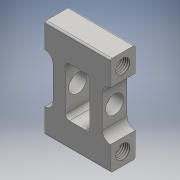
# Autodesk Inventor part: Profile_Middle_04
Saved by Autodesk Inventor 2016 (Build 200138000, 138)
## iProperties
Created: 2016-02-09
Part Number: Profile_Middle_04
Material: Generic
Document SubType Name: Modeling
Designer: nils
Density: 1 g/cm^3
Appearance: Default
Mass: 151.957 g
Surface Area: 392.667 cm^2
Volume: 151.957 cm^3
Author: nils
Autodesk Inventor part; units mm, degrees
ref_plane "YZ Plane" through (0, 0, 0) normal (1, 0, 0) x (0, 1, 0)
ref_plane "XZ Plane" through (0, 0, 0) normal (0, 1, 0) x (-1, 0, 0)
sketch "Sketch1" plane through (0, 0, 0) normal (1, 0, 0) x (0, 1, 0)
  line L0 (-15, 60) -> (15, 60)
  line L1 (15, 60) -> (15, -60)
  line L2 (15, -60) -> (-15, -60)
  line L3 (-15, -60) -> (-15, 60)
  line L4 (-15, 60) -> (15, -60) construction
  line L5 (15, 60) -> (-15, -60) construction
  point P0 (0, 0)
  dimension "d0" = 30
  dimension "d1" = 120
  constraints: 12 end point, 2 midpoint, 2 parallel, 1 horizontal, 1 perpendicular
  measures "d0" distance of L1.end L2.end
  measures "d1" distance of L0.end L1.end
extrude "Extrusion1" add sketch "Sketch1" along normal blind 80
sketch "Sketch2" plane through (80, 0, 0) normal (1, 0, 0) x (0, 0, -1)
  line L0 (-60, 15) -> (-60, -15) projected
  line L1 (-60, 0) -> (60, 0)
  line L2 (60, -15) -> (60, 15) projected
  line L3 (60, 15) -> (-60, 15) projected
  line L4 (0, 15) -> (0, -15)
  line L5 (-60, -15) -> (60, -15) projected
  point P0 (0, 0)
  point P1 (-45, 0)
  point P2 (45, 0)
  dimension "d4" = 45
  constraints: 4 end point, 4 midpoint, 2 point on line, 1 symmetric about line
  measures "d4" distance from line of L4 point (-45, 0)
hole "Hole1" at (80, 0, 45) at (80, 0, -45) direction (-1, 0, 0) diameter 17.294 depth 41.2 tip angle 118 thread size "M20x2.5" class "6H" standard "ISO Metric profile"
ref_plane "Work Plane1" through (40, 0, 0) normal (1, 0, 0) x (0, 0, -1)
mirror "Mirror1" about plane through (40, 0, 0) normal (1, 0, 0) of "Hole1"
sketch "Sketch5" plane through (0, 15, 60) normal (0, 1, 0) x (1, 0, 0)
  line L0 (0, 0) -> (80, 0) projected
  line L1 (40, 0) -> (40, 120)
  line L2 (0, 120) -> (80, 120) projected
  line L3 (55, 30) -> (25, 30)
  line L4 (25, 30) -> (25, 90)
  line L5 (25, 90) -> (55, 90)
  line L6 (55, 90) -> (55, 30)
  line L7 (55, 30) -> (25, 90) construction
  line L8 (25, 30) -> (55, 90) construction
  line L9 (0, 0) -> (0, 120) projected
  line L10 (0, 30) -> (10, 30)
  line L11 (10, 30) -> (10, 90)
  line L12 (10, 90) -> (0, 90)
  line L13 (0, 90) -> (0, 30)
  line L14 (80, 0) -> (80, 120) projected
  line L15 (80, 30) -> (70, 30)
  line L16 (70, 30) -> (70, 90)
  line L17 (70, 90) -> (80, 90)
  line L18 (80, 90) -> (80, 30)
  point P0 (0, 60)
  point P1 (40, 60)
  dimension "d20" = 30
  dimension "d22" = 30
  dimension "d23" = 30
  dimension "d24" = 60
  dimension "d25" = 10
  dimension "d26" = 10
  constraints: 30 end point, 6 parallel, 5 midpoint, 4 point on line, 3 horizontal, 3 perpendicular, 1 collinear
  measures "d20" distance between parallel lines of L0 L3
  measures "d22" distance between parallel lines of L6 L4
  measures "d23" distance between parallel lines of L2 L5
  measures "d24" distance between parallel lines of L17 L15
  measures "d25" distance between parallel lines of L18 L16
  measures "d26" distance between parallel lines of L9 L11
extrude "Extrusion2" cut sketch "Sketch5" against normal through all contours L9 L12 L11 L10 | L3 L4 L5 L1 | L1 L5 L6 L3 | L15 L16 L17 L14
hole "Hole5" at (70, 0, 0) direction (-1, 0, 0) diameter 22 end through all
fillet "Fillet1" radius 2 4 edges at (40, 15, 60) (40, -15, 60) (40, -15, -60) (40, 15, -60)
fillet "Fillet4" radius 10 2 edges at (70, 0, 30) (10, 0, 30)
fillet "Fillet5" radius 5 2 edges at (25, 0, 30) (55, 0, 30)
fillet "Fillet6" radius 10 2 edges at (70, 0, -30) (10, 0, -30)
fillet "Fillet9" radius 5 2 edges at (25, 0, -30) (55, 0, -30)
body "Solid1"
